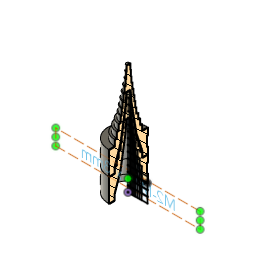
metric-hole-cones-v10 (Autodesk Fusion 360 design; units mm, degrees)
Autodesk Fusion 360 part; units mm, degrees
sketch "M2-M14 Profile Stacking" plane through (0, 0, 0) normal (0, 1, 0) x (1, 0, 0)
  line L0 (0, -18) -> (5, -18)
  line L1 (5, -18) -> (5, -21)
  line L2 (5, -21) -> (0, -21)
  line L3 (0, -21) -> (0, -18)
  line L4 (0, -21) -> (4, -21)
  line L5 (4, -21) -> (4, -24)
  line L6 (4, -24) -> (0, -24)
  line L7 (0, -24) -> (0, -21)
  line L8 (0, -24) -> (3.5, -24)
  line L9 (3.5, -24) -> (3.5, -27)
  line L10 (3.5, -27) -> (0, -27)
  line L11 (0, -27) -> (0, -24)
  line L12 (0, -27) -> (3, -27)
  line L13 (3, -27) -> (3, -30)
  line L14 (3, -30) -> (0, -30)
  line L15 (0, -30) -> (0, -27)
  line L16 (0, -30) -> (2.5, -30)
  line L17 (2.5, -30) -> (2.5, -33)
  line L18 (2.5, -33) -> (0, -33)
  line L19 (0, -33) -> (0, -30)
  line L20 (0, -33) -> (2, -33)
  line L21 (2, -33) -> (2, -36)
  line L22 (2, -36) -> (0, -36)
  line L23 (0, -36) -> (0, -33)
  line L24 (0, -36) -> (1.5, -36)
  line L25 (1.5, -36) -> (1.5, -39)
  line L26 (1.5, -39) -> (0, -39)
  line L27 (0, -39) -> (0, -36)
  line L28 (0, -39) -> (1.25, -39)
  line L29 (1.25, -39) -> (1.25, -42)
  line L30 (1.25, -42) -> (0, -42)
  line L31 (0, -42) -> (0, -39)
  line L32 (0, -42) -> (1, -42)
  line L33 (1, -42) -> (1, -45)
  line L34 (1, -45) -> (0, -45)
  line L35 (0, -45) -> (0, -42)
  line L36 (1, -42) -> (1, 0)
  line L37 (1.25, -39) -> (1.25, 0)
  line L38 (1.5, -36) -> (1.5, 0)
  line L39 (2, -33) -> (2, 0)
  line L40 (2.5, -30) -> (2.5, 0)
  line L41 (3, -27) -> (3, 0)
  line L42 (3.5, -24) -> (3.5, 0)
  line L43 (0, -18) -> (6, -18)
  line L44 (6, -18) -> (6, -15)
  line L45 (6, -15) -> (0, -15)
  line L46 (0, -15) -> (0, -18)
  line L47 (0, -15) -> (7, -15)
  line L48 (6, -15) -> (6, 0)
  line L49 (4, -21) -> (4, 0)
  line L50 (5, -18) -> (5, 0)
  line L51 (0, 0) -> (0, -3)
  line L52 (4, -12) -> (3.5, -15)
  line L53 (3.5, -15) -> (3, -18)
  line L54 (3, -18) -> (2.5, -21)
  line L55 (2.5, -21) -> (2, -24)
  line L56 (2, -24) -> (1.5, -27)
  line L57 (1.5, -27) -> (1.25, -30)
  line L58 (1.25, -30) -> (1, -33)
  line L59 (0, 0) -> (10, 0)
  line L60 (10, 0) -> (10, -3)
  line L61 (10, -3) -> (0, -3)
  line L62 (0, -3) -> (10, -3)
  line L63 (10, -3) -> (10, -6)
  line L64 (10, -6) -> (0, -6)
  line L65 (0, -6) -> (0, -3)
  line L66 (0, -6) -> (10, -6)
  line L67 (10, -6) -> (10, -9)
  line L68 (10, -9) -> (0, -9)
  line L69 (0, -9) -> (0, -6)
  line L70 (0, -9) -> (10, -9)
  line L71 (7, -15) -> (7, 0)
  line L72 (7, -3) -> (6, -6)
  line L73 (6, -6) -> (5, -9)
  line L74 (0, -9) -> (10, -9)
  line L75 (10, -9) -> (10, -12)
  line L76 (10, -12) -> (0, -12)
  line L77 (0, -12) -> (0, -9)
  line L78 (0, -12) -> (7, -12)
  line L79 (7, -12) -> (7, -15)
  line L80 (0, -15) -> (0, -12)
  line L81 (4, -12) -> (5, -9)
  line L82 (-37, -1.9991) -> (37, -1.9991) construction
  line L83 (37, -1.9991) -> (37, -10.0009) construction
  line L84 (37, -10.0009) -> (-37, -10.0009) construction
  line L85 (-37, -10.0009) -> (-37, -1.9991) construction
  dimension "d91" = 5
  dimension "d92" = 3
  dimension "d93" = 4
  dimension "d94" = 3
  dimension "d95" = 3.5
  dimension "d96" = 3
  dimension "d97" = 3
  dimension "d98" = 3
  dimension "d99" = 2.5
  dimension "d100" = 3
  dimension "d101" = 2
  dimension "d102" = 3
  dimension "d103" = 1.5
  dimension "d104" = 3
  dimension "d105" = 1.25
  dimension "d106" = 3
  dimension "d107" = 1
  dimension "d108" = 3
  dimension "d143" = 6
  dimension "d144" = 3
  dimension "d158" = 10
  dimension "d159" = 3
  dimension "d160" = 10
  dimension "d161" = 3
  dimension "d162" = 10
  dimension "d163" = 3
  dimension "d164" = 10
  dimension "d172" = 10
  dimension "d173" = 3
  dimension "d174" = 3
  dimension "d175" = 7
  dimension "d176" = 5
  text T0 "M2-M14 x 3mm" font "Arial" height 5 align centre middle in box 74 x 8.0018 at (-37, -1.9991) x (1, 0) y (0, -1) spacing 1 mirrored across
  constraint horizontal L0
  constraint vertical L1
  constraint horizontal L2
  constraint vertical L3
  constraint horizontal L4
  constraint vertical L5
  constraint horizontal L6
  constraint vertical L7
  constraint horizontal L8
  constraint vertical L9
  constraint horizontal L10
  constraint vertical L11
  constraint horizontal L12
  constraint vertical L13
  constraint horizontal L14
  constraint vertical L15
  constraint horizontal L16
  constraint vertical L17
  constraint horizontal L18
  constraint vertical L19
  constraint horizontal L20
  constraint vertical L21
  constraint horizontal L22
  constraint vertical L23
  constraint horizontal L24
  constraint vertical L25
  constraint horizontal L26
  constraint vertical L27
  constraint horizontal L28
  constraint vertical L29
  constraint horizontal L30
  constraint vertical L31
  constraint horizontal L32
  constraint vertical L33
  constraint horizontal L34
  constraint vertical L35
  constraint horizontal L43
  constraint vertical L44
  constraint horizontal L45
  constraint vertical L46
  constraint horizontal L47
  constraint vertical L51
  constraint coincident L49 L52.start
  constraint midpoint L47 L52.end
  constraint midpoint L43 L53.end
  constraint midpoint L2 L54.end
  constraint midpoint L6 L55.end
  constraint midpoint L12 L56.end
  constraint midpoint L16 L57.end
  constraint midpoint L20 L58.end
  constraint horizontal L59
  constraint vertical L60
  constraint horizontal L61
  constraint horizontal L62
  constraint vertical L63
  constraint horizontal L64
  constraint vertical L65
  constraint horizontal L66
  constraint vertical L67
  constraint horizontal L68
  constraint vertical L69
  constraint horizontal L70
  constraint coincident L51.end L61.end
  constraint coincident L51.start L59.start
  constraint vertical L36
  constraint vertical L37
  constraint vertical L38
  constraint vertical L39
  constraint vertical L40
  constraint vertical L41
  constraint vertical L42
  constraint vertical L49
  constraint vertical L50
  constraint vertical L48
  constraint coincident L36.end L59
  constraint coincident L37.end L59
  constraint coincident L39.end L59
  constraint coincident L40.end L59
  constraint midpoint L50.end L59
  constraint coincident L48.end L59
  constraint coincident L59 L71.end
  constraint perpendicular L59 L71
  constraint midpoint L73.end L68
  constraint coincident L62 L72.start
  constraint coincident L71 L72.start
  constraint coincident L48 L72.end
  constraint coincident L64 L72.end
  constraint coincident L38.end L59
  constraint coincident L42.end L59
  constraint coincident L41.end L59
  constraint coincident L49.end L59
  constraint horizontal L74
  constraint vertical L75
  constraint horizontal L76
  constraint vertical L77
  constraint horizontal L78
  constraint vertical L79
  constraint vertical L80
  constraint coincident L45.end L46.start
  constraint midpoint L73.end L70
  constraint coincident L52.start L78
  constraint horizontal L82
  constraint coincident L64.end
  measures "d91" distance of L0.start L0.end
  measures "d92" distance of L0.start L2.end
  measures "d93" distance of L2.end L4.end
  measures "d94" distance of L2.end L6.end
  measures "d95" distance of L6.end L8.end
  measures "d96" distance of L6.end L10.end
  measures "d97" distance of L10.end L12.end
  measures "d98" distance of L10.end L14.end
  measures "d99" distance of L14.end L16.end
  measures "d100" distance of L14.end L18.end
  measures "d101" distance of L18.end L20.end
  measures "d102" distance of L18.end L22.end
  measures "d103" distance of L22.end L24.end
  measures "d104" distance of L22.end L26.end
  measures "d105" distance of L26.end L28.end
  measures "d106" distance of L26.end L30.end
  measures "d107" distance of L30.end L32.end
  measures "d108" distance of L30.end L34.end
  measures "d143" distance of L0.start L43.end
  measures "d144" distance of L0.start L45.end
  measures "d158" distance of L51.start L59.end
  measures "d159" distance of L51.start L51.end
  measures "d160" distance of L51.end L60.end
  measures "d161" distance of L51.end L64.end
  measures "d162" distance of L64.end L63.end
  measures "d163" distance of L64.end L68.end
  measures "d164" distance of L68.end L67.end
  measures "d172" distance of L68.end L67.end
  measures "d173" distance of L68.end L76.end
  measures "d174" distance of L76.end L45.end
  measures "d175" distance of L79 L80
revolve "Revolve6" add sketch "M2-M14 Profile Stacking" angle 360 about axis through (0, 0, 0) along (0, 0, 1) contours L18 L20 L22 L23 L24 L36 | L0 L42 L43 L53 | L0 L2 L4 L41 L42 L43 | L2 L4 L41 L54 | L2 L4 L6 L8 L40 L41 | L6 L8 L40 L55 | L6 L8 L10 L12 L39 L40 | L10 L12 L39 L56 | L10 L12 L14 L16 L38 L39 | L14 L16 L38 L57 | L14 L16 L18 L20 L37 L38 | L18 L20 L37 L58 | L18 L20 L22 L24 L36 L37 | L22 L24 L26 L27 L28 L36 | L0 L42 L43 L45 L47 L49 | L0 L2 L4 L42 L43 L49 | L2 L4 L6 L8 L41 L42 | L45 L47 L49 L52 | L6 L8 L10 L12 L40 L41 | L10 L12 L14 L16 L39 L40 | L14 L16 L18 L20 L38 L39 | L18 L20 L22 L24 L37 L38 | L22 L24 L26 L28 L36 L37 | L26 L28 L30 L31 L32 L36 | L0 L43 L45 L47 L49 L50 | L0 L1 L2 L43 L49 | L2 L4 L5 L6 L42 | L6 L8 L9 L10 L41 | L45 L47 L49 L50 L76 L78 | L50 L76 L78 L81 | L10 L12 L13 L14 L40 | L14 L16 L17 L18 L39 | L18 L20 L21 L22 L38 | L22 L24 L25 L26 L37 | L26 L28 L29 L30 L36 | L30 L32 L33 L34 L35 | L43 L44 L45 L47 L50 | L45 L47 L48 L50 L76 L78 | L48 L50 L68 L70 L74 L76 L78 | L48 L68 L70 L73 L74 | L47 L48 L71 L76 L78 L79 | L48 L68 L70 L71 L74 L76 L78 | L48 L64 L66 L68 L70 L71 L74 | L64 L66 L71 L72 | L68 L70 L71 L74 L75 L76 | L64 L66 L67 L68 L70 L71 L74 | L61 L62 L63 L64 L66 L71 | L59 L60 L61 L62 L71 makes body 1
copy_body "Body->Comp7" bodies 1 removing the originals makes body 2 in component "M2-M14"
move_face "OffsetFaces1" offset -0.1 8 faces at (-0.4445, -1.1326, 30.4) (-2.4247, -3.0405, 12.6667) (6.9913, -0.3489, 2) (-0.1301, 0.6963, 33) (-2.4356, -6.2058, 4) (-2.0703, -5.275, 7) (4.3046, -2.073, 9.6667) (-0.7002, -1.7842, 24.5) on bodies 2 in component "M2-M14"
emboss "Emboss1" depth -0.5 profiles "M2-M14 Profile Stacking" section 1 text T0 onto face at (9.9503, -0.9957, 2) on bodies 2 bodies 2 in component "M2-M14"
component "M2-M14" placed x (1, 0, 0) y (0, 1, 0) z (0, 0, 1) at (0, 0, 0)
component "M2-M14" placed x (1, 0, 0) y (0, 1, 0) z (0, 0, 1) at (0, 0, 12)
equation "stack_height = 3 mm"
equation "d92 = stack_height"
equation "d94 = stack_height"
equation "d96 = stack_height"
equation "d98 = stack_height"
equation "d100 = stack_height"
equation "d102 = stack_height"
equation "d104 = stack_height"
equation "d105 = ( 2.5 / 2 ) * 1 mm"
equation "d106 = stack_height"
equation "d108 = stack_height"
equation "base_dia = 20 mm"
equation "d144 = stack_height"
equation "d159 = stack_height"
equation "d160 = base_dia / 2"
equation "d161 = stack_height"
equation "d162 = base_dia / 2"
equation "d163 = stack_height"
equation "d164 = base_dia / 2"
equation "d172 = base_dia / 2"
equation "d173 = stack_height"
equation "d174 = stack_height"
